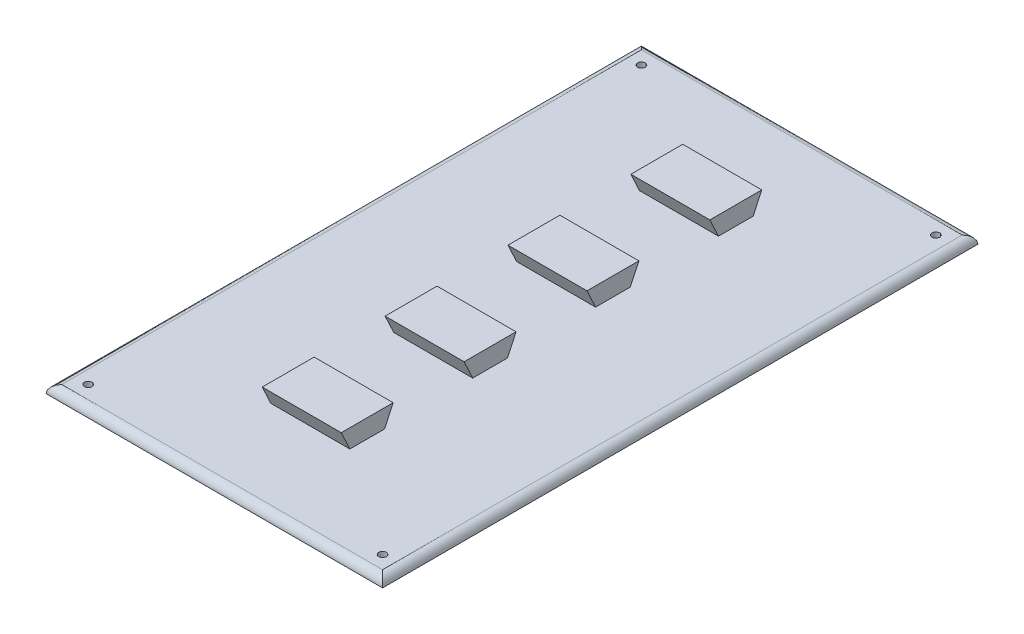
# Autodesk Inventor part: Lid
Saved by Autodesk Inventor 2023 (Build 270158000, 158)
## iProperties
Created: 2023-01-17
Part Number: Lid
Material: Generic
Document SubType Name: Modeling
Designer: Ahmed Nazir
Density: 1 g/cm^3
Appearance: Default
Author: Ahmed Nazir
Autodesk Inventor part; units mm, degrees
ref_plane "XZ Plane" through (0, 0, 0) normal (0, 1, 0) x (-1, 0, 0)
ref_plane "XY Plane" through (0, 0, 0) normal (0, 0, 1) x (1, 0, 0)
sketch "Sketch1" plane through (0, 0, 0) normal (0, 1, 0) x (-1, 0, 0)
  line L0 (0, 0) -> (-127.76, 0)
  line L1 (-127.76, 0) -> (-127.76, -226)
  line L2 (-127.76, -226) -> (0, -226)
  line L3 (0, -226) -> (0, 0)
  line L4 (-3, -3) -> (-124.76, -3)
  line L5 (-124.76, -3) -> (-124.76, -223)
  line L6 (-124.76, -223) -> (-3, -223)
  line L7 (-3, -223) -> (-3, -3)
  dimension "d0" = 127.76
  dimension "d1" = 226
  dimension "d2" = 3
  constraints: 16 end point, 4 parallel, 2 perpendicular, 1 horizontal, 3 other
  measures "d0" distance of L2.end L1.end
  measures "d1" distance of L1.end L0.end
  measures "d2" distance between parallel lines of L3 L7
extrude "Extrusion1" add sketch "Sketch1" against normal blind 3 contours L7 L6 L5 L4
extrude "Extrusion2" add sketch "Sketch1" along normal blind 3 contours L3 L2 L1 L0 | L7 L6 L5 L4
sketch "Sketch2" plane through (0, 3, 0) normal (0, 1, 0) x (1, 0, 0)
  line L0 (0, 226) -> (0, 0) projected
  line L1 (0, 113) -> (127.76, 113) construction
  line L2 (127.76, 0) -> (127.76, 226) projected
  line L3 (0, 0) -> (127.76, 0) projected
  line L4 (63.88, 0) -> (63.88, 226) construction
  line L5 (127.76, 226) -> (0, 226) projected
  circle A0 centre (119.76, 8) radius 1.5
  circle A1 centre (8, 8) radius 1.5
  circle A2 centre (119.76, 218) radius 1.5
  circle A3 centre (8, 218) radius 1.5
  dimension "d7" = 3
  dimension "d8" = 8
  dimension "d9" = 8
  constraints: 4 centre point, 4 end point, 4 midpoint, 3 symmetric about line, 3 other
  measures "d7" diameter of A0
  measures "d8" distance from line of L2 A0.centre
  measures "d9" distance from line of L3 A0.centre
extrude "Extrusion3" cut sketch "Sketch2" against normal through all contours A0 | A1 | A2 | A3
fillet "Fillet1" radius 3 4 edges at (127.76, 3, -113) (63.88, 3, -226) (0, 3, -113) (63.88, 3, 0)
ref_plane "Work Plane1" through (63.88, 0, 0) normal (1, 0, 0) x (0, 1, 0)
sketch "Sketch3" plane through (63.88, 0, 0) normal (1, 0, 0) x (0, 1, 0)
  line L0 (3, -223) -> (3, -3) projected
  line L1 (3, -49.634) -> (3, -36.46)
  line L2 (3, -36.46) -> (10, -33.1958)
  line L3 (10, -33.1958) -> (10, -52.8982)
  line L4 (10, -52.8982) -> (3, -49.634)
  line L5 (3, -96.268) -> (3, -83.094)
  line L6 (3, -83.094) -> (10, -79.8298)
  line L7 (10, -99.5322) -> (3, -96.268)
  line L8 (10, -99.5322) -> (10, -79.8298)
  arc A0 (0, -226) -> (3, -223) centre (0, -223) ccw projected
  line L9 (3, -223) -> (3, -3)
  line L10 (3, -113) -> (30.6964, -113) construction
  line L11 (3, -176.366) -> (3, -189.54)
  line L12 (3, -189.54) -> (10, -192.8042)
  line L13 (10, -192.8042) -> (10, -173.1018)
  line L14 (10, -173.1018) -> (3, -176.366)
  line L15 (3, -129.732) -> (3, -142.906)
  line L16 (3, -142.906) -> (10, -146.1702)
  line L17 (10, -126.4678) -> (3, -129.732)
  line L18 (10, -126.4678) -> (10, -146.1702)
  point P0 (0, 0)
  point P1 (3, -129.732)
  point P2 (3, -176.366)
  dimension "d14" = 13.174
  dimension "d15" = 65
  dimension "d16" = 65
  dimension "d17" = 7
  dimension "d18" = 33.46
  dimension "d19" = 13.174
  dimension "d20" = 33.46
  dimension "d22" = 65
  dimension "d23" = 65
  dimension "d24" = 7
  constraints: 36 end point, 8 symmetric about line, 4 point on line, 2 vertical, 1 collinear, 1 horizontal, 1 midpoint, 1 tangent
  measures "d14" distance of L1.start L1.end
  measures "d15" angle of L0 L4
  measures "d16" angle of L0 L2
  measures "d17" distance between parallel lines of L0 L3
  measures "d18" distance of L0.end L1.end
  measures "d19" distance of L5.start L5.end
  measures "d20" distance of L1.start L5.end
  measures "d22" angle of L0 L6
  measures "d23" angle of L0 L7
  measures "d24" distance between parallel lines of L0 L8
extrude "Extrusion4" add sketch "Sketch3" along normal mid plane 30
body "Solid1"
